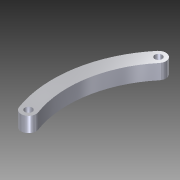
# Autodesk Inventor part: ledeplate
Saved by Autodesk Inventor 2015 (Build 190159000, 159)
## iProperties
Created: 2015-02-05
Part Number: ledeplate
Material: Generic
Document SubType Name: Modeling
Designer: janov_000
Density: 1 g/cm^3
Appearance: Aluminum - Flat
Author: janov_000
Autodesk Inventor part; units mm, degrees
ref_plane "YZ Plane" through (0, 0, 0) normal (1, 0, 0) x (0, 1, 0)
ref_plane "XZ Plane" through (0, 0, 0) normal (0, 1, 0) x (-1, 0, 0)
ref_plane "XY Plane" through (0, 0, 0) normal (0, 0, 1) x (1, 0, 0)
sketch "Sketch1" plane through (0, 0, 0) normal (0, 0, 1) x (1, 0, 0)
  arc A0 (-154.1048, 152.1451) -> (-166.8784, 78.2408) centre (-96.4886, 104.1307) ccw construction
  arc A1 (-157.9458, 155.346) -> (-171.571, 76.5148) centre (-96.4886, 104.1307) ccw
  arc A2 (-150.2637, 148.9441) -> (-162.1857, 79.9668) centre (-96.4886, 104.1307) ccw
  arc A3 (-150.2637, 148.9441) -> (-157.9458, 155.346) centre (-154.1048, 152.1451) ccw
  arc A4 (-171.571, 76.5148) -> (-162.1857, 79.9668) centre (-166.8784, 78.2408) ccw
  line L0 (-154.1048, 152.1451) -> (-96.4886, 104.1307) construction
  line L1 (-96.4886, 104.1307) -> (-166.8784, 78.2408) construction
  point P0 (0, 0)
  dimension "d1" = 75
  dimension "d2" = 10
  dimension "d5" = 60
  constraints: 10 point on circle, 5 centre point, 4 end point, 4 tangent, 1 coincident
  measures "d1" radius of A0
  measures "d2" diameter of A3
  measures "d5" angle of L1 L0
extrude "Extrusion1" add sketch "Sketch1" along normal blind 10
sketch "Sketch2" plane through (0, 0, 10) normal (0, 0, 1) x (1, 0, 0)
  arc A0 (-157.9458, 155.346) -> (-171.571, 76.5148) centre (-96.4886, 104.1307) ccw projected
  arc A1 (-171.571, 76.5148) -> (-162.1857, 79.9668) centre (-166.8784, 78.2408) ccw projected
  arc A2 (-150.2637, 148.9441) -> (-162.1857, 79.9668) centre (-96.4886, 104.1307) ccw projected
  arc A3 (-150.2637, 148.9441) -> (-157.9458, 155.346) centre (-154.1048, 152.1451) ccw projected
  point P0 (0, 0)
  constraints: 2 coincident
hole "Hole1" at (-154.1048, 152.1451, 10) at (-166.8784, 78.2408, 10) direction (0, 0, -1) diameter 5 end through all
body "Solid1"
